servo_slide (Autodesk Fusion 360 design; units mm, degrees)
Autodesk Fusion 360 part; units mm, degrees
sketch "Sketch1" plane through (0, 0, 0) normal (0, 0, 1) x (1, 0, 0)
sketch "Sketch2" plane through (0, 0, 4) normal (0, 0, 1) x (-1, 0, 0)
  line L0 (-20, 1.25) -> (0, 1.25)
  arc A0 (0, -1.25) -> (0, 1.25) centre (0, 0) ccw
  line L1 (0, -1.25) -> (-20, -1.25)
  arc A1 (-20, 1.25) -> (-20, -1.25) centre (-20, 0) ccw
  line L2 (6, 4.25) -> (-26, 4.25)
  line L3 (-26, 4.25) -> (-26, 2.25)
  arc A2 (-26, 2.25) -> (-25, 1.25) centre (-25, 2.25) ccw
  line L4 (-25, 1.25) -> (-25.244, 1.25)
  arc A3 (-24.2452, 0.2024) -> (-25.244, 1.25) centre (-25.244, 0.25) ccw
  arc A4 (-24.2452, 0.2024) -> (-20, -4.25) centre (-20, 0) ccw
  line L5 (-20, -4.25) -> (0, -4.25)
  arc A5 (0, -4.25) -> (4.244, 0.2261) centre (0, 0) ccw
  arc A6 (5.2426, 1.2793) -> (4.244, 0.2261) centre (5.2426, 0.2793) ccw
  line L6 (5.2426, 1.2793) -> (5, 1.2793)
  arc A7 (5, 1.2793) -> (6, 2.2793) centre (5, 2.2793) ccw
  line L7 (6, 2.2793) -> (6, 4.25)
  line L8 (-75, -1.25) -> (-45, -1.25)
  arc A8 (-45, -1.25) -> (-45, 1.25) centre (-45, 0) ccw
  line L9 (-45, 1.25) -> (-75, 1.25)
  arc A9 (-75, 1.25) -> (-75, -1.25) centre (-75, 0) ccw
  line L10 (-75, 0) -> (-45, 0) construction
  line L11 (-45, 4.25) -> (-75, 4.25)
  arc A10 (-79.2452, 0.2024) -> (-75, -4.25) centre (-75, 0) ccw
  line L12 (-75, -4.25) -> (-45, -4.25)
  arc A11 (-45, -4.25) -> (-40.7548, 0.2024) centre (-45, 0) ccw
  line L13 (-75, 4.25) -> (-81, 4.25)
  line L14 (-81, 4.25) -> (-81, 2.25)
  line L15 (-80, 1.25) -> (-80.244, 1.25)
  line L16 (-45, 4.25) -> (-39, 4.25)
  line L17 (-39, 4.25) -> (-39, 2.25)
  line L18 (-40, 1.25) -> (-39.756, 1.25)
  arc A12 (-39.756, 1.25) -> (-40.7548, 0.2024) centre (-39.756, 0.25) ccw
  arc A13 (-40, 1.25) -> (-39, 2.25) centre (-40, 2.25) ccw
  arc A14 (-81, 2.25) -> (-80, 1.25) centre (-80, 2.25) ccw
  arc A15 (-79.2452, 0.2024) -> (-80.244, 1.25) centre (-80.244, 0.25) ccw
  dimension "d24" = 2.5
  dimension "d26" = 6
  dimension "d28" = 6
  dimension "d30" = 1
  dimension "d31" = 1
  dimension "d32" = 1
  dimension "d33" = 1
  constraint tangent L8 A8
  constraint tangent A8 L9
  constraint parallel L8 L9
  constraint tangent L9 A9
  constraint tangent L8 A9
  constraint horizontal L10
  constraint horizontal L13
  constraint vertical L14
  constraint horizontal L15
  constraint horizontal L16
  constraint vertical L17
  constraint horizontal L18
  constraint concentric A9 A10
  constraint concentric A8 A11
  constraint tangent L11 A11
  constraint tangent L12 A11
  constraint tangent L11 A10
  constraint tangent A10 L12
  constraint tangent L18 A12
  constraint tangent A11 A12
  constraint tangent L17 A13
  constraint tangent L18 A13
  constraint tangent L15 A14
  constraint tangent L14 A14
  constraint tangent A10 A15
  constraint tangent L15 A15
  measures "d24" diameter of A8
  measures "d26" distance of L11.end L13.end
  measures "d28" distance of L11.start L16.end
  measures "d30" radius of A12
  measures "d31" radius of A13
  measures "d32" radius of A14
  measures "d33" radius of A15
sketch "Sketch3" plane through (0, 0, 8) normal (0, 0, 1) x (-1, 0, 0)
  arc A0 (-75, 1.25) -> (-75, -1.25) centre (-75, 0) ccw
  line L0 (-75, 1.25) -> (-45, 1.25)
  arc A1 (-45, -1.25) -> (-45, 1.25) centre (-45, 0) ccw
  line L1 (-45, -1.25) -> (-75, -1.25)
  line L2 (-75, -4.25) -> (-45, -4.25)
  arc A2 (-45, -4.25) -> (-40.7548, 0.2024) centre (-45, 0) ccw
  arc A3 (-39.756, 1.25) -> (-40.7548, 0.2024) centre (-39.756, 0.25) ccw
  line L3 (-39.756, 1.25) -> (-40, 1.25)
  arc A4 (-40, 1.25) -> (-39, 2.25) centre (-40, 2.25) ccw
  line L4 (-39, 2.25) -> (-39, 4.25)
  line L5 (-39, 4.25) -> (-81, 4.25)
  line L6 (-81, 4.25) -> (-81, 2.25)
  arc A5 (-81, 2.25) -> (-80, 1.25) centre (-80, 2.25) ccw
  line L7 (-80, 1.25) -> (-80.244, 1.25)
  arc A6 (-79.2452, 0.2024) -> (-80.244, 1.25) centre (-80.244, 0.25) ccw
  arc A7 (-79.2452, 0.2024) -> (-75, -4.25) centre (-75, 0) ccw
  line L8 (-78, 13.75) -> (-48, 13.75)
  arc A8 (-48, 13.75) -> (-48, 16.25) centre (-48, 15) ccw
  line L9 (-48, 16.25) -> (-78, 16.25)
  arc A9 (-78, 16.25) -> (-78, 13.75) centre (-78, 15) ccw
  line L10 (-78, 15) -> (-48, 15) construction
  line L11 (-48, 19.25) -> (-78, 19.25)
  arc A10 (-82.2452, 15.2024) -> (-78, 10.75) centre (-78, 15) ccw
  line L12 (-78, 10.75) -> (-48, 10.75)
  arc A11 (-48, 10.75) -> (-43.7548, 15.2024) centre (-48, 15) ccw
  line L13 (-48, 19.25) -> (-42, 19.25)
  line L14 (-42, 19.25) -> (-42, 16.75)
  line L15 (-42.5, 16.25) -> (-42.756, 16.25)
  line L16 (-78, 19.25) -> (-84, 19.25)
  line L17 (-84, 19.25) -> (-84, 16.75)
  line L18 (-83.5, 16.25) -> (-83.244, 16.25)
  arc A12 (-42.756, 16.25) -> (-43.7548, 15.2024) centre (-42.756, 15.25) ccw
  arc A13 (-42.5, 16.25) -> (-42, 16.75) centre (-42.5, 16.75) ccw
  arc A14 (-82.2452, 15.2024) -> (-83.244, 16.25) centre (-83.244, 15.25) ccw
  arc A15 (-84, 16.75) -> (-83.5, 16.25) centre (-83.5, 16.75) ccw
  dimension "d36" = 2.5
  dimension "d38" = 6
  dimension "d40" = 6
  dimension "d42" = 1
  dimension "d43" = 0.5
  dimension "d44" = 1
  dimension "d45" = 0.5
  constraint tangent L8 A8
  constraint tangent A8 L9
  constraint parallel L8 L9
  constraint tangent L9 A9
  constraint tangent L8 A9
  constraint horizontal L10
  constraint horizontal L13
  constraint vertical L14
  constraint horizontal L15
  constraint horizontal L16
  constraint vertical L17
  constraint horizontal L18
  constraint concentric A9 A10
  constraint concentric A8 A11
  constraint tangent L11 A11
  constraint tangent L11 A10
  constraint tangent L12 A11
  constraint tangent A10 L12
  constraint tangent A11 A12
  constraint tangent L15 A12
  constraint tangent L14 A13
  constraint tangent L15 A13
  constraint tangent A10 A14
  constraint tangent L18 A14
  constraint tangent L17 A15
  constraint tangent L18 A15
  measures "d36" diameter of A8
  measures "d38" distance of L11.start L13.end
  measures "d40" distance of L11.end L16.end
  measures "d42" radius of A12
  measures "d43" radius of A13
  measures "d44" radius of A14
  measures "d45" radius of A15
extrude "Extrude3" add sketch "Sketch3" along normal blind 4 contours L11 A10 L12 A11 L13 L14 L15 L16 L17 L18 A12 A13 A14 A15 makes body 1
sketch "Sketch4" plane through (0, 0, 0) normal (0, 0, 1) x (1, 0, 0)
  line L0 (0, -16.25) -> (20, -16.25)
  arc A0 (20, -16.25) -> (20, -13.75) centre (20, -15) ccw
  line L1 (20, -13.75) -> (0, -13.75)
  arc A1 (0, -13.75) -> (0, -16.25) centre (0, -15) ccw
  line L2 (0, -15) -> (20, -15) construction
  line L3 (0, -19.25) -> (20, -19.25)
  arc A2 (24.2452, -15.2024) -> (20, -10.75) centre (20, -15) ccw
  line L4 (20, -10.75) -> (0, -10.75)
  arc A3 (0, -10.75) -> (-4.2452, -15.2024) centre (0, -15) ccw
  line L5 (0, -19.25) -> (-6, -19.25)
  line L6 (-6, -19.25) -> (-6, -16.75)
  line L7 (-5.5, -16.25) -> (-5.244, -16.25)
  line L8 (20, -19.25) -> (26, -19.25)
  line L9 (26, -19.25) -> (26, -16.75)
  line L10 (25.5, -16.25) -> (25.244, -16.25)
  arc A4 (24.2452, -15.2024) -> (25.244, -16.25) centre (25.244, -15.25) ccw
  arc A5 (-5.244, -16.25) -> (-4.2452, -15.2024) centre (-5.244, -15.25) ccw
  arc A6 (26, -16.75) -> (25.5, -16.25) centre (25.5, -16.75) ccw
  arc A7 (-5.5, -16.25) -> (-6, -16.75) centre (-5.5, -16.75) ccw
  dimension "d48" = 2.5
  dimension "d50" = 6
  dimension "d52" = 6
  dimension "d54" = 1
  dimension "d55" = 1
  dimension "d56" = 0.5
  dimension "d57" = 0.5
  constraint tangent L0 A0
  constraint tangent A0 L1
  constraint parallel L0 L1
  constraint tangent L1 A1
  constraint tangent L0 A1
  constraint horizontal L2
  constraint horizontal L5
  constraint vertical L6
  constraint horizontal L7
  constraint horizontal L8
  constraint vertical L9
  constraint horizontal L10
  constraint concentric A0 A2
  constraint concentric A1 A3
  constraint tangent L3 A3
  constraint tangent L3 A2
  constraint tangent A2 L4
  constraint tangent L4 A3
  constraint tangent A2 A4
  constraint tangent L10 A4
  constraint tangent A3 A5
  constraint tangent L7 A5
  constraint tangent L9 A6
  constraint tangent L10 A6
  constraint tangent L6 A7
  constraint tangent L7 A7
  measures "d48" diameter of A0
  measures "d50" distance of L3.start L5.end
  measures "d52" distance of L3.end L8.end
  measures "d54" radius of A4
  measures "d55" radius of A5
  measures "d56" radius of A6
  measures "d57" radius of A7
extrude "Extrude4" add sketch "Sketch4" along normal blind 4 separate body makes body 2
